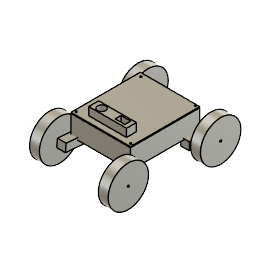
SensBot v3 (Autodesk Fusion 360 design; units mm, degrees)
Autodesk Fusion 360 part; units mm, degrees
sketch "Sketch1" plane through (0, 0, 0) normal (0, 1, 0) x (1, 0, 0)
  line L0 (0, 0) -> (300, 0)
  line L1 (300, 0) -> (300, 350)
  line L2 (300, 350) -> (0, 350)
  line L3 (0, 350) -> (0, 0)
  dimension "d1" = 300
  dimension "d2" = 350
  constraint horizontal L0
  constraint vertical L1
  constraint horizontal L2
  constraint vertical L3
  constraint coincident L0.start L3.end
  measures "d1" distance of L0.start L0.end
  measures "d2" distance of L0.start L2.end
extrude "Extrude1" add sketch "Sketch1" along normal blind 100 makes body 1
sketch "Sketch2" plane through (0, 100, 0) normal (0, 1, 0) x (-1, 0, 0)
  line L0 (0, -350) -> (0, 0)
  line L1 (0, 0) -> (-300, 0)
  line L2 (-300, 0) -> (-300, -350)
  line L3 (-300, -350) -> (0, -350)
  line L4 (-22.1021, -22.1021) -> (-277.8979, -22.1021)
  line L5 (-277.8979, -22.1021) -> (-277.8979, -327.8979)
  line L6 (-277.8979, -327.8979) -> (-22.1021, -327.8979)
  line L7 (-22.1021, -327.8979) -> (-22.1021, -22.1021)
  dimension "d5" = -22.1021
extrude "Extrude2" cut sketch "Sketch2" against normal blind 82 contours L4 L5 L6 L7 bodies 1
sketch "Sketch3" plane through (0, 0, 0) normal (0, 1, 0) x (1, 0, 0)
  line L0 (-470, 0) -> (-170, 0)
  line L1 (-170, 0) -> (-170, -350)
  line L2 (-170, -350) -> (-470, -350)
  line L3 (-470, -350) -> (-470, 0)
  dimension "d8" = 300
  dimension "d9" = 350
  constraint horizontal L0
  constraint vertical L1
  constraint horizontal L2
  constraint vertical L3
  measures "d8" distance of L0.start L0.end
  measures "d9" distance of L0.start L2.end
extrude "Extrude3" add sketch "Sketch3" along normal blind 5 separate body makes body 2
move_body "Move1" bodies 2 to x (1, 0, 0) y (0, 1, 0) z (0, 0, 1) at (470, 100, -350)
sketch "Sketch4" plane through (0, 105, 0) normal (0, 1, 0) x (-1, 0, 0)
  line L0 (0, 0) -> (-300, 0)
  line L1 (-300, 0) -> (-300, -350)
  line L2 (-300, -350) -> (0, -350)
  line L3 (0, -350) -> (0, 0)
  line L4 (-273.4489, -26.5511) -> (-273.4489, -323.4489)
  line L5 (-273.4489, -323.4489) -> (-26.5511, -323.4489)
  line L6 (-26.5511, -323.4489) -> (-26.5511, -26.5511)
  line L7 (-26.5511, -26.5511) -> (-273.4489, -26.5511)
  line L8 (-15.0433, -15.0433) -> (-11.5078, -11.5078)
  circle A0 centre (-13.2756, -13.2756) radius 2.5
  line L9 (-284.9567, -15.0433) -> (-288.4922, -11.5078)
  circle A1 centre (-286.7244, -13.2756) radius 2.5
  dimension "d12" = -26.5511
  dimension "d13" = 5
  dimension "d14" = 5
  dimension "d15" = 26.5511
  constraint coincident A0 L8.start
  constraint coincident L8 A0.centre
  constraint coincident A0 L8.end
  constraint coincident A1 L9.start
  constraint coincident L9 A1.centre
  constraint coincident A1 L9.end
  measures "d13" diameter of A0
  measures "d14" diameter of A1
  measures "d15" distance of L3 L6.end
extrude "Extrude4" cut sketch "Sketch4" against normal blind 10 contours L8 A0 | L8 A0 bodies 1 2
sketch "Sketch5" plane through (0, 105, 0) normal (0, 1, 0) x (-1, 0, 0)
  circle A0 centre (-13.2756, -13.2756) radius 2.5
  line L0 (0, 0) -> (-300, 0)
  line L1 (-300, 0) -> (-300, -350)
  line L2 (-300, -350) -> (0, -350)
  line L3 (0, -350) -> (0, 0)
  circle A1 centre (-287.6495, -13.2756) radius 2.5
  line L4 (-13.2756, -13.2756) -> (-15.7756, -13.2756)
  line L5 (-285.1495, -13.2756) -> (-290.1495, -13.2756)
  dimension "d18" = 5
  constraint coincident A0.centre L4.start
  constraint perpendicular L1 L4
  constraint coincident A1.centre L4
  constraint coincident A0 L4.end
  constraint coincident A1 L5.start
  constraint collinear L4 L5
  constraint coincident A1 L5.end
  measures "d18" diameter of A1
extrude "Extrude5" cut sketch "Sketch5" against normal blind 10 contours A1 L5 | A1 L5 bodies 1 2
sketch "Sketch6" plane through (0, 105, 0) normal (0, 1, 0) x (-1, 0, 0)
  circle A0 centre (-287.6495, -13.2756) radius 2.5
  circle A1 centre (-13.2756, -13.2756) radius 2.5
  line L0 (0, 0) -> (-300, 0)
  line L1 (-300, 0) -> (-300, -350)
  line L2 (-300, -350) -> (0, -350)
  line L3 (0, -350) -> (0, 0)
  circle A2 centre (-288.0052, -340.1367) radius 2.5
  dimension "d21" = 5
  measures "d21" diameter of A2
extrude "Extrude6" cut sketch "Sketch6" against normal blind 10 contours A2 bodies 1 2
sketch "Sketch7" plane through (0, 105, 0) normal (0, 1, 0) x (-1, 0, 0)
  circle A0 centre (-288.0052, -340.1367) radius 2.5
  circle A1 centre (-287.6495, -13.2756) radius 2.5
  circle A2 centre (-13.2756, -13.2756) radius 2.5
  line L0 (0, 0) -> (-300, 0)
  line L1 (-300, 0) -> (-300, -350)
  line L2 (-300, -350) -> (0, -350)
  line L3 (0, -350) -> (0, 0)
  circle A3 centre (-22.7529, -330.2226) radius 2.5
  dimension "d24" = 5
  measures "d24" diameter of A3
extrude "Extrude7" cut sketch "Sketch7" against normal blind 10 contours A3 bodies 1 2
sketch "Sketch8" plane through (0, 0, 0) normal (0, 1, 0) x (1, 0, 0)
  line L0 (60, 80, 105) -> (60, 30, 105)
  line L1 (60, 30, 105) -> (250, 30, 105)
  line L2 (250, 30, 105) -> (250, 80, 105)
  line L3 (250, 80, 105) -> (60, 80, 105)
  line L4 (60, 80, 105) -> (250, 80, 105)
  line L5 (250, 80, 105) -> (250, 30, 105)
  line L6 (250, 30, 105) -> (60, 30, 105)
  line L7 (60, 30, 105) -> (60, 80, 105)
extrude "Extrude8" add sketch "Sketch8" along normal blind 40 contours L0 L1 L2 L3 L4 L5 L6 L7 in plane through (0, 105, 0) normal (0, 1, 0) bodies 2
sketch "Sketch9" plane through (0, 145, 0) normal (0, 1, 0) x (-1, 0, 0)
  line L0 (-60, -30) -> (-250, -30)
  line L1 (-250, -30) -> (-250, -80)
  line L2 (-250, -80) -> (-60, -80)
  line L3 (-60, -80) -> (-60, -30)
  circle A0 centre (-99.8069, -55) radius 20.5393
  line L4 (-176.4327, -67.3779) -> (-216.789, -67.3779)
  line L5 (-216.789, -67.3779) -> (-216.789, -42.8577)
  line L6 (-216.789, -42.8577) -> (-176.4327, -42.8577)
  line L7 (-176.4327, -42.8577) -> (-176.4327, -67.3779)
  constraint horizontal L4
  constraint vertical L5
  constraint horizontal L6
  constraint vertical L7
extrude "Extrude9" cut sketch "Sketch9" against normal blind 75 contours A0 bodies 2
sketch "Sketch10" plane through (0, 145, 0) normal (0, 1, 0) x (-1, 0, 0)
  circle A0 centre (-99.8069, -55) radius 20.5393
  line L0 (-60, -30) -> (-250, -30)
  line L1 (-250, -30) -> (-250, -80)
  line L2 (-250, -80) -> (-60, -80)
  line L3 (-60, -80) -> (-60, -30)
  line L4 (-180.4786, -72.1698) -> (-229.1247, -72.1698)
  line L5 (-229.1247, -72.1698) -> (-229.1247, -42.9822)
  line L6 (-229.1247, -42.9822) -> (-180.4786, -42.9822)
  line L7 (-180.4786, -42.9822) -> (-180.4786, -72.1698)
  constraint horizontal L4
  constraint vertical L5
  constraint horizontal L6
  constraint vertical L7
extrude "Extrude10" cut sketch "Sketch10" against normal blind 75 contours L4 L5 L6 L7 bodies 2
sketch "Sketch11" plane through (0, 0, 0) normal (0, 1, 0) x (1, 0, 0)
  circle A0 centre (-186.9136, 50.8036) radius 4
  dimension "d33" = 8
  measures "d33" diameter of A0
extrude "Extrude11" add sketch "Sketch11" along normal blind 2 separate body makes body 3
sketch "Sketch12" plane through (0, 2, 0) normal (0, 1, 0) x (-1, 0, 0)
  circle A0 centre (186.9136, -50.8036) radius 4
  circle A1 centre (186.9136, -50.8036) radius 2.5
  dimension "d36" = 5
  constraint concentric A0 A1
  measures "d36" diameter of A1
extrude "Extrude12" add sketch "Sketch12" along normal blind 10 contours A1 bodies 3
thread "Thread1" "ISO Metric profile 5.0 M5x0.8 M5x0.8 6g" major diameter 4.901 minor diameter 3.9895 pitch 0.8 angle 60 resizes the face on face at (-187.5907, 8.6667, -48.397) on bodies 3
copy_body "CopyPasteBodies1" bodies 3 makes body 4
move_body "Move2" bodies 4 to x (1, 0, 0) y (0, 1, 0) z (0, 0, 1) at (22, 0, 0)
copy_body "CopyPasteBodies2" bodies 3 makes body 5
move_body "Move3" bodies 5 to x (1, 0, 0) y (0, 1, 0) z (0, 0, 1) at (0, 31, 0)
copy_body "CopyPasteBodies3" bodies 3 makes body 6
move_body "Move4" bodies 6 to x (1, 0, 0) y (0, 1, 0) z (0, 0, 1) at (0, 0, 19)
move_body "Move5" bodies 4 to x (-1, 0, 0) y (0, -1, 0) z (0, 0, 1) at (-153.917, 107, 36.2209)
move_body "Move6" bodies 6 to x (1, 0, 0) y (0, -1, 0) z (0, 0, -1) at (475.8322, 108, -44.6068)
move_body "Move7" bodies 3 to x (1, 0, 0) y (0, -1, 0) z (0, 0, -1) at (210.2106, 108.8359, -380.6332)
move_body "Move8" bodies 5 to x (-1, 0, 0) y (0, -1, 0) z (0, 0, 1) at (100.8268, 140.0617, -289.4056)
sketch "Sketch13" plane through (0, 0, 0) normal (0, 1, 0) x (1, 0, 0)
  line L0 (-140.7781, -56.2396) -> (-20, -56.2396)
  line L1 (-20, -56.2396) -> (-20, -100)
  line L2 (-20, -100) -> (-140.7781, -100)
  line L3 (-140.7781, -100) -> (-140.7781, -56.2396)
  constraint horizontal L0
  constraint vertical L1
  constraint horizontal L2
  constraint vertical L3
extrude "Extrude13" add sketch "Sketch13" along normal blind 40 separate body makes body 7
sketch "Sketch14" plane through (0, 0, 100) normal (0, 0, 1) x (1, 0, 0)
  line L0 (-140.7781, 0) -> (-20, 0)
  line L1 (-20, 0) -> (-20, 40)
  line L2 (-20, 40) -> (-140.7781, 40)
  line L3 (-140.7781, 40) -> (-140.7781, 0)
  circle A0 centre (-120, 20) radius 5
  dimension "d43" = 10
  measures "d43" diameter of A0
extrude "Extrude14" add sketch "Sketch14" along normal blind 30 contours A0 bodies 7
sketch "Sketch15" plane through (0, 40, 0) normal (0, 1, 0) x (-1, 0, 0)
  line L0 (140.7781, 100) -> (20, 100)
  line L1 (20, 100) -> (20, 56.2396)
  line L2 (20, 56.2396) -> (140.7781, 56.2396)
  line L3 (140.7781, 56.2396) -> (140.7781, 100)
sketch "Sketch16" plane through (0, 0, 0) normal (0, 0, 1) x (1, 0, 0)
  circle A0 centre (-345.6064, 10.7165) radius 102.06
extrude "Extrude15" add sketch "Sketch16" along normal blind 50 separate body makes body 8
sketch "Sketch17" plane through (0, 0, 50) normal (0, 0, 1) x (1, 0, 0)
  circle A0 centre (-345.6064, 10.7165) radius 102.06
  circle A1 centre (-345.6064, 10.7165) radius 5
  dimension "d48" = 10
  constraint concentric A0 A1
  measures "d48" diameter of A1
hole "Hole1" at (-345.6064, 10.7165, 50) direction (0, 0, -1) diameter 10 depth 125 tip angle 118 bodies 8
move_body "Move9" bodies 8 to x (1, 0, 0) y (0, 1, 0) z (0, 0, 1) at (224.4136, 7.7921, 106.757)
move_body "Move10" bodies 8 7 to x (1, 0, 0) y (0, 1, 0) z (0, 0, 1) at (-46.9575, -27.7892, 132.1333)
copy_body "CopyPasteBodies4" bodies 8 7 makes body 9 makes body 10
move_body "Move11" bodies 9 10 to x (1, 0, 0) y (0, 1, 0) z (0, 0, 1) at (178.202, -154.3531, 77.1357)
copy_body "CopyPasteBodies5" bodies 8 7 makes body 11 makes body 12
move_body "Move12" bodies 11 12 to x (1, 0, 0) y (0, 1, 0) z (0, 0, 1) at (166.1814, -129.3876, -208.3837)
copy_body "CopyPasteBodies6" bodies 8 7 makes body 13 makes body 14
move_body "Move13" bodies 13 14 to x (1, 0, 0) y (0, 1, 0) z (0, 0, 1) at (20.4338, 170.4129, -145.6052)
move_body "Move14" bodies 14 13 to x (-0.001329, -0.015134, -0.999885) y (0.000651, 0.999885, -0.015134) z (0.999999, -0.000671, -0.001319) at (216.2959, -166.3622, -74.9687)
move_body "Move15" bodies 12 11 to x (0, -0.087156, -0.996195) y (0, -0.996195, 0.087156) z (-1, 0, 0) at (13.9788, -142.2793, 50.5668)
move_body "Move16" bodies 9 10 to x (0, 0, 1) y (0, 1, 0) z (-1, 0, 0) at (304.6991, 151.1106, -410.288)
move_body "Move17" bodies 7 8 to x (0, 0, 1) y (0, -1, 0) z (1, 0, 0) at (97.4716, -21.1099, -200.8659)
